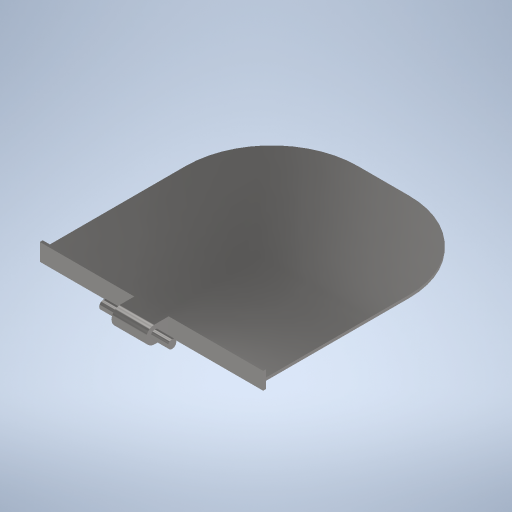
# Autodesk Inventor part: aperature_panel
Saved by Autodesk Inventor 2024 (Build 280153000, 153)
## iProperties
Created: 2024-04-15
Part Number: aperature_panel
Material: Stainless Steel AISI 440C, Welded
Document SubType Name: Modeling
Designer: soham
Density: 7.8 g/cm^3
Appearance: Steel - Polished
Author: soham
Autodesk Inventor part; units mm, degrees
ref_plane "YZ Plane" through (0, 0, 0) normal (1, 0, 0) x (0, 1, 0)
ref_plane "XZ Plane" through (0, 0, 0) normal (0, 1, 0) x (-1, 0, 0)
ref_plane "XY Plane" through (0, 0, 0) normal (0, 0, 1) x (1, 0, 0)
sketch "panel_sketch" plane through (0, 0, 0) normal (0, 1, 0) x (-1, 0, 0)
  line L0 (195, 0) -> (195, -250)
  line L1 (195, 0) -> (0, 0)
  line L2 (0, 0) -> (0, -400)
  line L3 (0, -400) -> (45, -400)
  arc A0 (45, -400) -> (195, -250) centre (45, -250) ccw
  line L4 (-195, 0) -> (-195, -250)
  line L5 (-195, 0) -> (0, 0)
  line L6 (0, -400) -> (-45, -400)
  arc A1 (-195, -250) -> (-45, -400) centre (-45, -250) ccw
  dimension "d1" = 400
  dimension "d2" = 390
  dimension "d3" = 250
  dimension "d4" = 45
  constraints: 14 end point, 4 point on circle, 4 symmetric about line, 2 centre point, 2 horizontal, 2 vertical, 1 tangent, 1 other
  measures "d1" distance of L1.end L2.end
  measures "d2" diameter of L0 L2
  measures "d3" distance of L0.start L0.end
  measures "d4" distance of L2.end L3.end
extrude "panel_extrude" add sketch "panel_sketch" along normal mid plane 5
sketch "hinge_sketch" plane through (0, 0, 0) normal (0, 1, 0) x (-1, 0, 0)
  line L0 (195, -250) -> (195, 0) projected
  line L1 (195, 0) -> (195, 5)
  line L2 (195, 5) -> (30, 5)
  line L3 (30, 5) -> (30, 45)
  line L4 (0, 0) -> (0, 150)
  line L5 (195, 0) -> (0, 0)
  line L6 (195, 0) -> (-195, 0) projected
  line L7 (30, 45) -> (0, 45)
  line L8 (-195, 0) -> (-195, 5)
  line L9 (-195, 5) -> (-30, 5)
  line L10 (-30, 5) -> (-30, 45)
  line L11 (-195, 0) -> (0, 0)
  line L12 (-30, 45) -> (0, 45)
  dimension "d8" = 5
  dimension "d9" = 60
  dimension "d10" = 40
  dimension "d19" = 150
  constraints: 22 end point, 3 symmetric about line, 2 perpendicular, 2 vertical, 1 collinear, 1 horizontal, 1 point on line
  measures "d8" distance of L0.end L1.end
  measures "d9" diameter of L3 L4
  measures "d10" distance of L2.end L3.end
  measures "d19" distance of L4.start L4.end
extrude "hinge_extrude" add sketch "hinge_sketch" along normal mid plane 30
fillet "hinge_bottom_fillet" radius 15 2 edges at (0, 15, 45) (0, -15, 45)
sketch "hinge_link_sketch" plane through (-30, -15, 5) normal (-1, 0, 0) x (0, 0, 1)
  line L0 (0, 30) -> (25, 30) projected
  arc A0 (25, 0) -> (25, 30) centre (25, 15) ccw projected
  line L1 (25, 0) -> (0, 0) projected
  circle A1 centre (24, 15) radius 7.5
  point P0 (-5, 15)
  point P1 (40, 15)
  dimension "d14" = 15
  dimension "d15" = 16
  dimension "d16" = 15
  constraints: 1 centre point, 1 point on circle
  measures "d14" diameter of A1
  measures "d15" distance of point (40, 15) A1.centre
  measures "d16" distance from line of L0 A1.centre
extrude "hinge_link_extrude" add sketch "hinge_link_sketch" along normal blind 30
mirror "hinge_link_extrude_mirror" about plane through (0, 0, 0) normal (1, 0, 0)
equation "\"d1\" = panel_height"
equation "\"d2\" = panel_width"
equation "\"d3\" = vertical_height"
equation "\"d4\" = 0.5 * panel_width + vertical_height - panel_height"
equation "\"d9\" = hinge_width"
equation "\"d10\" = hinge_height"
equation "\"d11\" = 0.5 * hinge_width"
equation "\"d17\" = 0.5 * hinge_width"
equation "\"panel_height\" = 400"
equation "\"panel_width\" = 390"
equation "\"vertical_height\" = 250"
equation "\"hinge_width\" = 60"
equation "\"hinge_height\" = 40"
body "Solid1"
